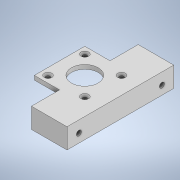
# Autodesk Inventor part: shoulder motor support
Saved by Autodesk Inventor 2022 (Build 260153000, 153)
## iProperties
Created: 2022-03-24
Part Number: shoulder motor support
Material: Genérico
Document SubType Name: Modeling
Designer: JK
Density: 1 g/cm^3
Appearance: Valor por defecto
Author: JK
Autodesk Inventor part; units mm, degrees
ref_plane "YZ Plane" through (0, 0, 0) normal (1, 0, 0) x (0, 1, 0)
ref_plane "XZ Plane" through (0, 0, 0) normal (0, 1, 0) x (-1, 0, 0)
ref_plane "XY Plane" through (0, 0, 0) normal (0, 0, 1) x (1, 0, 0)
sketch "Boceto1" plane through (0, 0, 0) normal (0, 1, 0) x (-1, 0, 0)
  circle A0 centre (0, 0) radius 11.25
  line L0 (-21.25, 21.25) -> (21.25, 21.25)
  line L1 (21.25, 21.25) -> (21.25, -21.25)
  line L2 (21.25, -21.25) -> (-21.25, -21.25)
  line L3 (-21.25, -21.25) -> (-21.25, 21.25)
  line L4 (-21.25, 21.25) -> (21.25, -21.25) construction
  line L5 (21.25, 21.25) -> (-21.25, -21.25) construction
  dimension "d0" = 22.5
  dimension "d1" = 42.5
  dimension "d2" = 42.5
  constraints: 12 end point, 2 midpoint, 2 parallel, 1 centre point, 1 coincident, 1 horizontal, 1 perpendicular
  measures "d0" diameter of A0
  measures "d1" distance of L0.end L1.end
  measures "d2" distance of L1.end L2.end
extrude "Extrusión1" add sketch "Boceto1" along normal blind 3.5
sketch "Boceto2" plane through (0, 3.5, 0) normal (0, 1, 0) x (1, 0, 0)
  circle A0 centre (-15.5, -15.5) radius 1.7
  point P0 (0, 0)
  dimension "d5" = 15.5
  dimension "d6" = 15.5
  dimension "d7" = 3.4
  constraints: 1 centre point
  measures "d5" horizontal distance of A0.centre point (0, 0)
  measures "d6" horizontal distance of A0.centre point (0, 0)
  measures "d7" diameter of A0
extrude "Extrusión2" cut sketch "Boceto2" against normal through all
chamfer "Chaflán1" distance 1.5 angle 45 1 edges at (-17.2, 3.5, 15.5)
pattern_circular "Patrón circular1" count 4 over 360 about axis through (0, 0, 0) along (0, 1, 0) of "Extrusión2", "Chaflán1"
sketch "Boceto3" plane through (0, 3.5, 0) normal (0, 1, 0) x (1, 0, 0)
  circle A0 centre (15.5, 15.5) radius 3.2 projected
  circle A1 centre (-15.5, -15.5) radius 3.2 projected
  line L0 (21.25, 21.25) -> (-21.25, 21.25) projected
  line L1 (-21.25, 21.25) -> (-21.25, -21.25) projected
  line L2 (-21.25, -21.25) -> (21.25, -21.25) projected
  line L3 (21.25, -21.25) -> (21.25, 21.25) projected
  circle A2 centre (0, 0) radius 11.25 projected
  circle A3 centre (15.5, -15.5) radius 3.2 projected
  circle A4 centre (-15.5, 15.5) radius 3.2 projected
  line L4 (0, -45) -> (30, -45)
  line L5 (30, -45) -> (30, 45)
  line L6 (30, 45) -> (0, 45)
  line L7 (0, 45) -> (0, -45)
  point P0 (0, -21.25)
  point P1 (0, 21.25)
  dimension "d16" = 90
  dimension "d17" = 45
  dimension "d18" = 0
  dimension "d19" = 30
  constraints: 8 end point, 2 parallel, 1 horizontal, 1 perpendicular
  measures "d16" distance between parallel lines of L6 L4
  measures "d17" distance from line of A2.centre L4
  measures "d18" distance from line of A2.centre L7
  measures "d19" distance between parallel lines of L7 L5
extrude "Extrusión3" add sketch "Boceto3" against normal blind 17 contours L0 L7 L6 L5 L4 L2 L3
sketch "Boceto4" plane through (30, 3.5, 45) normal (1, 0, 0) x (0, 0, -1)
  circle A0 centre (10, -9.65) radius 2.1 projected
  circle A1 centre (80, -9.65) radius 2.1 projected
  point P0 (45, -3.5)
extrude "Extrusión4" cut sketch "Boceto4" against normal through all
